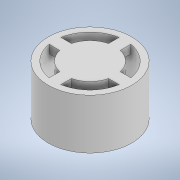
# Autodesk Inventor part: Wheel
Saved by Autodesk Inventor 2020.1 (Build 241239000, 239)
## iProperties
Created: 2019-11-14
Part Number: Wheel
Material: Generic
Document SubType Name: Modeling
Designer: super
Density: 1 g/cm^3
Appearance: Default
Author: super
Autodesk Inventor part; units mm, degrees
note: some values were not read from the file. Chosen so that the rebuilt part matches the saved one: second side of "Extrusion4".
ref_plane "YZ Plane" through (0, 0, 0) normal (1, 0, 0) x (0, 1, 0)
ref_plane "XZ Plane" through (0, 0, 0) normal (0, 1, 0) x (-1, 0, 0)
ref_plane "XY Plane" through (0, 0, 0) normal (0, 0, 1) x (1, 0, 0)
sketch "Sketch1" plane through (0, 0, 0) normal (0, 1, 0) x (-1, 0, 0)
  circle A0 centre (0, 0) radius 25
  dimension "d0" = 50
  constraints: 1 centre point, 1 coincident
  measures "d0" diameter of A0
extrude "Extrusion1" add sketch "Sketch1" along normal blind 30
sketch "Sketch2" plane through (0, 30, 0) normal (0, 1, 0) x (1, 0, 0)
  circle A0 centre (0, 0) radius 21.25
  dimension "d3" = 42.5
  constraints: 1 centre point, 1 coincident
  measures "d3" diameter of A0
extrude "Extrusion2" cut sketch "Sketch2" against normal blind 30
sketch "Sketch3" plane through (0, 30, 0) normal (0, 1, 0) x (1, 0, 0)
  circle A0 centre (0, 0) radius 15
  dimension "d6" = 30
  constraints: 1 centre point, 1 coincident
  measures "d6" diameter of A0
extrude "Extrusion3" add sketch "Sketch3" against normal blind 5
sketch "Sketch4" plane through (0, 30, 0) normal (0, 1, 0) x (1, 0, 0)
  circle A0 centre (0, 0) radius 21.25 projected
  line L0 (0, -12.25) -> (3.5, -12.25)
  line L1 (3.5, -12.25) -> (3.5, -22.5574)
  line L2 (3.5, -22.5574) -> (-3.5, -22.5574)
  line L3 (-3.5, -22.5574) -> (-3.5, -12.25)
  line L4 (-3.5, -12.25) -> (0, -12.25)
  point P0 (-3.5, -20.9598)
  point P1 (3.5, -20.9598)
  dimension "d10" = 3.5
  dimension "d11" = 7
  constraints: 10 end point, 3 perpendicular, 1 vertical
  measures "d10" distance of L0.start L0.end
  measures "d11" distance of L1.end L2.end
extrude "Extrusion4" add sketch "Sketch4" against normal blind 5 contours L3 L4 L0 L1 A0 picked at (1.5571, -15.2392)
sketch "Sketch5" plane through (0, 30, 0) normal (0, 1, 0) x (1, 0, 0)
  circle A0 centre (0, 0) radius 21.25 projected
  line L0 (12.1299, 0) -> (12.1299, 3.5)
  line L1 (12.1299, 3.5) -> (23.3023, 3.5)
  line L2 (23.3023, 3.5) -> (23.3023, -3.5)
  line L3 (23.3023, -3.5) -> (12.1299, -3.5)
  line L4 (12.1299, -3.5) -> (12.1299, 3.5)
  point P0 (20.9598, -3.5)
  point P1 (20.9598, 3.5)
  dimension "d16" = 3.5
  dimension "d17" = 7
  constraints: 10 end point, 4 perpendicular, 1 point on line
  measures "d16" distance of L0.start L0.end
  measures "d17" distance of L1.end L2.end
extrude "Extrusion5" add sketch "Sketch5" against normal blind 5 contours A0 L3 L4 L0 L1 picked at (15.1269, -1.9464)
sketch "Sketch6" plane through (0, 30, 0) normal (0, 1, 0) x (1, 0, 0)
  line L0 (0, 13.5132) -> (-3.5, 13.5132)
  line L1 (-3.5, 13.5132) -> (-3.5, 23.3023)
  line L2 (-3.5, 23.3023) -> (3.5, 23.3023)
  line L3 (3.5, 23.3023) -> (3.5, 13.5132)
  line L4 (3.5, 13.5132) -> (-3.5, 13.5132)
  point P0 (0, 0)
  dimension "d20" = 7
  constraints: 10 end point, 4 perpendicular, 1 horizontal, 1 point on line
  measures "d20" distance of L1.end L2.end
extrude "Extrusion6" add sketch "Sketch6" against normal blind 5
sketch "Sketch7" plane through (0, 30, 0) normal (0, 1, 0) x (1, 0, 0)
  line L0 (-12.9812, 0) -> (-12.9812, -3.5)
  line L1 (-12.9812, -3.5) -> (-22.5574, -3.5)
  line L2 (-22.5574, -3.5) -> (-22.5574, 3.5)
  line L3 (-22.5574, 3.5) -> (-12.9812, 3.5)
  line L4 (-12.9812, 3.5) -> (-12.9812, 0)
  point P0 (0, 0)
  dimension "d23" = 3.5
  dimension "d24" = 7
  constraints: 10 end point, 3 perpendicular, 1 collinear, 1 point on line, 1 vertical
  measures "d23" distance of L0.start L0.end
  measures "d24" distance of L1.end L2.end
extrude "Extrusion7" add sketch "Sketch7" against normal blind 5
sketch "Sketch8" plane through (0, 25, 0) normal (0, -1, 0) x (1, 0, 0)
  circle A0 centre (0, 0) radius 10
  dimension "d27" = 20
  constraints: 1 centre point, 1 coincident
  measures "d27" diameter of A0
extrude "Extrusion8" add sketch "Sketch8" along normal blind 20
sketch "Sketch9" plane through (0, 5, 0) normal (0, -1, 0) x (1, 0, 0)
  circle A0 centre (0, 0) radius 7.5
  dimension "d30" = 15
  constraints: 1 centre point, 1 coincident
  measures "d30" diameter of A0
extrude "Extrusion9" cut sketch "Sketch9" against normal blind 20
sketch "Sketch10" plane through (0, 0, 0) normal (0, -1, 0) x (1, 0, 0)
  circle A0 centre (0, 0) radius 15
  constraints: 1 centre point, 1 coincident
extrude "Extrusion10" add sketch "Sketch10" against normal blind 5
sketch "Sketch11" plane through (0, 0, 0) normal (0, -1, 0) x (1, 0, 0)
  line L0 (12.662, 0) -> (12.662, 3.5)
  line L1 (12.662, 3.5) -> (22.2382, 3.5)
  line L2 (22.2382, 3.5) -> (22.2382, -3.5)
  line L3 (22.2382, -3.5) -> (12.662, -3.5)
  line L4 (12.662, -3.5) -> (12.662, 0)
  point P0 (0, 0)
  dimension "d35" = 3.5
  dimension "d36" = 7
  constraints: 10 end point, 4 perpendicular, 1 point on line, 1 vertical
  measures "d35" distance of L0.start L0.end
  measures "d36" distance of L1.end L2.end
extrude "Extrusion11" add sketch "Sketch11" against normal blind 5
sketch "Sketch12" plane through (0, 0, 0) normal (0, -1, 0) x (1, 0, 0)
  line L0 (0, 12.3428) -> (3.5, 12.3428)
  line L1 (3.5, 12.3428) -> (3.5, 22.5574)
  line L2 (3.5, 22.5574) -> (-3.5, 22.5574)
  line L3 (-3.5, 22.5574) -> (-3.5, 12.3428)
  line L4 (-3.5, 12.3428) -> (0, 12.3428)
  point P0 (0, 0)
  dimension "d39" = 3.5
  dimension "d40" = 7
  constraints: 10 end point, 4 perpendicular, 1 horizontal, 1 point on line
  measures "d39" distance of L0.start L0.end
  measures "d40" distance of L1.end L2.end
extrude "Extrusion12" add sketch "Sketch12" against normal blind 5
sketch "Sketch13" plane through (0, 0, 0) normal (0, -1, 0) x (1, 0, 0)
  line L0 (0, -13.726) -> (3.5, -13.726)
  line L1 (3.5, -13.726) -> (3.5, -22.5574)
  line L2 (3.5, -22.5574) -> (-3.5, -22.5574)
  line L3 (-3.5, -22.5574) -> (-3.5, -13.726)
  line L4 (-3.5, -13.726) -> (0, -13.726)
  point P0 (0, 0)
  dimension "d43" = 3.5
  dimension "d44" = 7
  constraints: 10 end point, 4 perpendicular, 1 horizontal, 1 point on line
  measures "d43" distance of L0.start L0.end
  measures "d44" distance of L1.end L2.end
extrude "Extrusion13" add sketch "Sketch13" against normal blind 5
sketch "Sketch14" plane through (0, 0, 0) normal (0, -1, 0) x (1, 0, 0)
  line L0 (-12.0235, 0) -> (-12.0235, -3.5)
  line L1 (-12.0235, -3.5) -> (-22.451, -3.5)
  line L2 (-22.451, -3.5) -> (-22.451, 3.5)
  line L3 (-22.451, 3.5) -> (-12.0235, 3.5)
  line L4 (-12.0235, 3.5) -> (-12.0235, 0)
  point P0 (0, 0)
  dimension "d47" = 3.5
  dimension "d48" = 7
  constraints: 10 end point, 4 perpendicular, 1 point on line, 1 vertical
  measures "d47" distance of L0.start L0.end
  measures "d48" distance of L1.end L2.end
extrude "Extrusion14" add sketch "Sketch14" against normal blind 5
body "Solid1"
